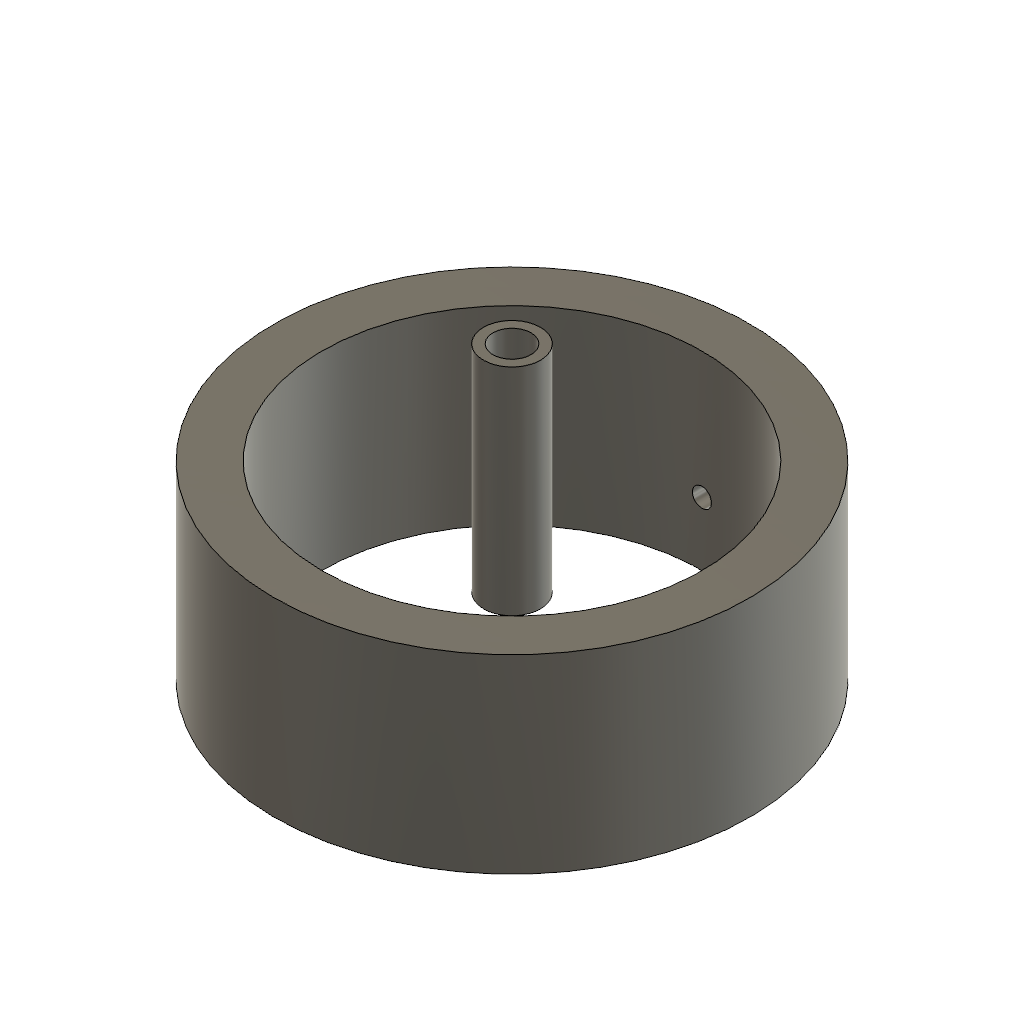
race tank (Autodesk Fusion 360 archive; units mm, degrees)
design "whel"
part number: 2026-05-14-16-49-29-881
Autodesk Fusion 360 part; units mm, degrees
sketch "Sketch1" plane through (0, 0, 0) normal (0, 1, 0) x (1, 0, 0)
  circle A0 centre (-9.0763, 7.4879) radius 42.5
  circle A1 centre (-9.0763, 7.4879) radius 30.0076
  line L0 (-13.6697, 40) -> (-4.7657, 40)
  line L1 (-4.7657, 40) -> (-4.7657, -24.506)
  line L2 (-4.7657, -24.506) -> (-13.6697, -24.506)
  line L3 (-13.6697, -24.506) -> (-13.6697, 40)
  line L4 (-41, 12.6264) -> (22, 12.6264)
  line L5 (22, 12.6264) -> (22, 3.3132)
  line L6 (22, 3.3132) -> (-41, 3.3132)
  line L7 (-41, 3.3132) -> (-41, 12.6264)
  line L8 (-9.0763, 7.4879) -> (-12.1102, 10.0947)
  line L9 (-9.0763, 7.4879) -> (-6.0424, 4.8812)
  line L10 (-12.1102, 10.0947) -> (-31.4914, -12.4624)
  line L11 (-6.0424, 4.8812) -> (-25.4235, -17.676)
  line L12 (-6.0424, 4.8812) -> (13.3388, 27.4383)
  line L13 (-12.1102, 10.0947) -> (7.2709, 32.6518)
  line L14 (-9.0763, 7.4879) -> (-6.4695, 10.5219)
  line L15 (-6.4695, 10.5219) -> (-29.0267, 29.903)
  line L16 (-6.4695, 10.5219) -> (16.0876, -8.8593)
  line L17 (-11.6831, 4.454) -> (10.8741, -14.9272)
  line L18 (-11.6831, 4.454) -> (-34.2402, 23.8352)
  dimension "d1" = 85
  dimension "d3" = 4
  dimension "d4" = 4
  dimension "d5" = 4
  dimension "d6" = 4
  constraint concentric A0 A1
  constraint horizontal L0
  constraint vertical L1
  constraint horizontal L2
  constraint vertical L3
  constraint horizontal L4
  constraint vertical L5
  constraint horizontal L6
  constraint vertical L7
  constraint coincident A0.centre A1.centre
  constraint parallel L8 L9
  constraint coincident A1 L10.end
  constraint perpendicular L8 L10
  constraint coincident A1 L11.end
  constraint perpendicular L9 L11
  constraint coincident A1 L12.end
  constraint perpendicular L9 L12
  constraint coincident A1 L13.end
  constraint perpendicular L8 L13
  constraint perpendicular L9 L14
  constraint coincident A1 L15.end
  constraint perpendicular L13 L15
  constraint coincident A1 L16.end
  constraint perpendicular L12 L16
  constraint coincident A1 L17.end
  constraint perpendicular L11 L17
  constraint coincident A1 L18.end
  measures "d1" diameter of A0
  measures "d3" distance of A0.centre L8.end
  measures "d4" distance of A0.centre L9.end
  measures "d5" distance of A0.centre L17.start
  measures "d6" distance of A0.centre L14.end
extrude "Extrude1" add sketch "Sketch1" along normal blind 40 contours A0 | A1 L1 L4 L12 L13 | A1 L4 L5 L6 | A1 L4 L6 L12 L16 | L1 L4 L12 L16 | A1 L1 L3 L13 L15 | A1 L0 L1 L3 | L1 L4 L13 L15 | L1 L4 L15 L16 | L1 L6 L12 L16 | L1 L12 L16 | L4 L13 L15 | L3 L4 L13 L15 | L1 L9 L12 L14 L16 | L4 L8 L13 L14 L15 | L1 L6 L11 L12 | A1 L1 L6 L16 L17 | A1 L3 L4 L15 L18 | L3 L4 L10 L13 | L1 L6 L11 L17 | L3 L6 L8 L9 L10 L11 L17 L18 | L3 L4 L10 L18 | A1 L1 L3 L11 L17 | L6 L11 L17 | A1 L4 L6 L10 L18 | A1 L4 L6 L7 | L3 L10 L18 | A1 L1 L2 L3 | L3 L6 L11 L17 | L3 L6 L17 L18 | L3 L6 L10 L18 | A1 L3 L6 L10 L11 makes body 1
sketch "Sketch2" plane through (0, 40, 0) normal (0, 1, 0) x (-1, 0, 0)
  circle A0 centre (9.0763, -7.4879) radius 42.5
  line L0 (-20.4881, -12.6264) -> (-0.6123, -12.6264)
  line L1 (-0.6123, -12.6264) -> (-13.3388, -27.4383)
  arc A1 (-20.4881, -12.6264) -> (-13.3388, -27.4383) centre (9.0763, -7.4879) ccw
  line L2 (-1.9204, -3.3132) -> (-20.6395, -3.3132)
  arc A2 (-16.0876, 8.8593) -> (-20.6395, -3.3132) centre (9.0763, -7.4879) ccw
  line L3 (-16.0876, 8.8593) -> (-1.9204, -3.3132)
  line L4 (4.7657, -18.6428) -> (4.7657, -37.1843)
  arc A3 (-7.2709, -32.6518) -> (4.7657, -37.1843) centre (9.0763, -7.4879) ccw
  line L5 (-7.2709, -32.6518) -> (4.7657, -18.6428)
  line L6 (13.6697, -37.1419) -> (13.6697, -16.7083)
  line L7 (13.6697, -16.7083) -> (29.0267, -29.903)
  arc A4 (13.6697, -37.1419) -> (29.0267, -29.903) centre (9.0763, -7.4879) ccw
  line L8 (21.1946, -12.6264) -> (38.6406, -12.6264)
  arc A5 (34.2402, -23.8352) -> (38.6406, -12.6264) centre (9.0763, -7.4879) ccw
  line L9 (34.2402, -23.8352) -> (21.1946, -12.6264)
  line L10 (13.6697, 3.996) -> (13.6697, 22.166)
  arc A6 (25.4235, 17.676) -> (13.6697, 22.166) centre (9.0763, -7.4879) ccw
  line L11 (25.4235, 17.676) -> (13.6697, 3.996)
  line L12 (4.7657, 22.2084) -> (4.7657, 1.4894)
  line L13 (4.7657, 1.4894) -> (-10.8741, 14.9272)
  arc A7 (4.7657, 22.2084) -> (-10.8741, 14.9272) centre (9.0763, -7.4879) ccw
  line L14 (38.792, -3.3132) -> (17.9369, -3.3132)
  line L15 (17.9369, -3.3132) -> (31.4914, 12.4624)
  arc A8 (38.792, -3.3132) -> (31.4914, 12.4624) centre (9.0763, -7.4879) ccw
  circle A9 centre (9.0763, -7.4879) radius 30.0076
  constraint concentric A0 A9
extrude "Extrude2" cut sketch "Sketch2" against normal blind 10 contours L0 L1 L2 L3 L4 L5 L6 L7 L8 L9 L10 L11 L12 L13 L14 L15 A9 bodies 1
sketch "Sketch3" plane through (0, 30, 0) normal (0, 1, 0) x (-1, 0, 0)
  arc A0 (38.6406, -12.6264) -> (38.792, -3.3132) centre (9.0763, -7.4879) ccw
  line L0 (38.792, -3.3132) -> (17.9369, -3.3132)
  line L1 (17.9369, -3.3132) -> (31.4914, 12.4624)
  arc A1 (31.4914, 12.4624) -> (25.4235, 17.676) centre (9.0763, -7.4879) ccw
  line L2 (25.4235, 17.676) -> (13.6697, 3.996)
  line L3 (13.6697, 3.996) -> (13.6697, 22.166)
  arc A2 (13.6697, 22.166) -> (4.7657, 22.2084) centre (9.0763, -7.4879) ccw
  line L4 (4.7657, 22.2084) -> (4.7657, 1.4894)
  line L5 (4.7657, 1.4894) -> (-10.8741, 14.9272)
  arc A3 (-10.8741, 14.9272) -> (-16.0876, 8.8593) centre (9.0763, -7.4879) ccw
  line L6 (-16.0876, 8.8593) -> (-1.9204, -3.3132)
  line L7 (-1.9204, -3.3132) -> (-20.6395, -3.3132)
  arc A4 (-20.6395, -3.3132) -> (-20.4881, -12.6264) centre (9.0763, -7.4879) ccw
  line L8 (-20.4881, -12.6264) -> (-0.6123, -12.6264)
  line L9 (-0.6123, -12.6264) -> (-13.3388, -27.4383)
  arc A5 (-13.3388, -27.4383) -> (-7.2709, -32.6518) centre (9.0763, -7.4879) ccw
  line L10 (-7.2709, -32.6518) -> (4.7657, -18.6428)
  line L11 (4.7657, -18.6428) -> (4.7657, -37.1843)
  arc A6 (4.7657, -37.1843) -> (13.6697, -37.1419) centre (9.0763, -7.4879) ccw
  line L12 (13.6697, -37.1419) -> (13.6697, -16.7083)
  line L13 (13.6697, -16.7083) -> (29.0267, -29.903)
  arc A7 (29.0267, -29.903) -> (34.2402, -23.8352) centre (9.0763, -7.4879) ccw
  line L14 (34.2402, -23.8352) -> (21.1946, -12.6264)
  line L15 (21.1946, -12.6264) -> (38.6406, -12.6264)
  circle A8 centre (9.0763, -7.4879) radius 6
  dimension "d11" = 12
  constraint concentric A0 A8
  measures "d11" diameter of A8
extrude "Extrude3" add sketch "Sketch3" along normal blind 20 contours A8 bodies 1
sketch "Sketch4" plane through (0, 50, 0) normal (0, 1, 0) x (-1, 0, 0)
  circle A0 centre (9.0763, -7.4879) radius 6
  circle A1 centre (9.0763, -7.4879) radius 3
  dimension "d14" = 6
  constraint concentric A0 A1
  measures "d14" diameter of A1
extrude "Extrude4" cut sketch "Sketch4" against normal blind 40 contours A1 bodies 1
move_face "MoveFace1" by (0, -10, 0) 1 faces at (-13.9891, 50, -8.2059) on bodies 1
move_face "MoveFace2" by (0, 10, 0) 1 faces at (-5.941, 0, -9.2817) on bodies 1
sketch "Sketch5" plane through (0, 10, 0) normal (0, -1, 0) x (1, 0, 0)
  line L0 (-17.9369, -3.3132) -> (-38.792, -3.3132)
  arc A0 (-31.4914, 12.4624) -> (-38.792, -3.3132) centre (-9.0763, -7.4879) ccw
  line L1 (-31.4914, 12.4624) -> (-17.9369, -3.3132)
  line L2 (-4.7657, 1.4894) -> (-4.7657, 22.2084)
  arc A1 (10.8741, 14.9272) -> (-4.7657, 22.2084) centre (-9.0763, -7.4879) ccw
  line L3 (10.8741, 14.9272) -> (-4.7657, 1.4894)
  line L4 (-13.6697, 22.166) -> (-13.6697, 3.996)
  line L5 (-13.6697, 3.996) -> (-25.4235, 17.676)
  arc A2 (-13.6697, 22.166) -> (-25.4235, 17.676) centre (-9.0763, -7.4879) ccw
  line L6 (-38.6406, -12.6264) -> (-21.1946, -12.6264)
  line L7 (-21.1946, -12.6264) -> (-34.2402, -23.8352)
  arc A3 (-38.6406, -12.6264) -> (-34.2402, -23.8352) centre (-9.0763, -7.4879) ccw
  line L8 (-13.6697, -16.7083) -> (-13.6697, -37.1419)
  arc A4 (-29.0267, -29.903) -> (-13.6697, -37.1419) centre (-9.0763, -7.4879) ccw
  line L9 (-29.0267, -29.903) -> (-13.6697, -16.7083)
  line L10 (-4.7657, -37.1843) -> (-4.7657, -18.6428)
  line L11 (-4.7657, -18.6428) -> (7.2709, -32.6518)
  arc A5 (-4.7657, -37.1843) -> (7.2709, -32.6518) centre (-9.0763, -7.4879) ccw
  line L12 (20.6395, -3.3132) -> (1.9204, -3.3132)
  line L13 (1.9204, -3.3132) -> (16.0876, 8.8593)
  arc A6 (20.6395, -3.3132) -> (16.0876, 8.8593) centre (-9.0763, -7.4879) ccw
  line L14 (0.6123, -12.6264) -> (20.4881, -12.6264)
  arc A7 (13.3388, -27.4383) -> (20.4881, -12.6264) centre (-9.0763, -7.4879) ccw
  line L15 (13.3388, -27.4383) -> (0.6123, -12.6264)
  circle A8 centre (-9.0763, -7.4879) radius 42.5
  circle A9 centre (-9.0763, -7.4879) radius 3
  circle A10 centre (-9.0763, -7.4879) radius 3
  circle A11 centre (-9.0763, -7.4879) radius 4.5
  dimension "d17" = 9
  constraint concentric A0 A10
  constraint concentric A0 A11
  measures "d17" diameter of A11
extrude "Extrude5" add sketch "Sketch5" along normal blind 10 separate body contours A11 makes body 2
sketch "Sketch6" plane through (0, 0, 0) normal (0, -1, 0) x (1, 0, 0)
  circle A0 centre (-9.0763, -7.4879) radius 3
  circle A1 centre (-9.0763, -7.4879) radius 4.5
  circle A2 centre (-9.0763, -7.4879) radius 4.5
  constraint concentric A0 A2
sketch "Sketch7" plane through (-2.7602, 0, 3.2125) normal (-0.651692, 0, 0.758484) x (0.758484, 0, 0.651692)
  line L0 (17.9757, 30) -> (-2.644, 30)
  line L1 (-2.644, 30) -> (-2.644, 10)
  line L2 (-2.644, 10) -> (17.9757, 10)
  line L3 (17.9757, 10) -> (17.9757, 30)
  line L4 (-11.7599, 0) -> (-11.7599, 6.7)
  line L5 (-11.7599, 0) -> (-11.7599, 9.4)
  line L6 (-11.7599, 6.7) -> (-11.7599, 8.05)
  line L7 (-11.7599, 0) -> (-11.7599, 10)
  circle A0 centre (-11.7599, 10) radius 1.5
  dimension "d21" = 6.7
  dimension "d22" = 9.4
  dimension "d23" = 1.35
  dimension "d34" = 3
  constraint parallel L4 L5
  constraint parallel L5 L6
  constraint parallel L5 L7
  constraint coincident L7.end A0.centre
  measures "d21" distance of L4.start L4.end
  measures "d22" distance of L4.start L5.end
  measures "d23" distance of L4.end L6.end
  measures "d34" diameter of A0
sketch "Sketch10" plane through (0, 10, 0) normal (0, -1, 0) x (1, 0, 0)
  circle A0 centre (-9.0763, -7.4879) radius 3
  circle A1 centre (-9.0763, -7.4879) radius 42.5
  line L0 (0.6123, -12.6264) -> (20.4881, -12.6264)
  arc A2 (13.3388, -27.4383) -> (20.4881, -12.6264) centre (-9.0763, -7.4879) ccw
  line L1 (13.3388, -27.4383) -> (0.6123, -12.6264)
  line L2 (20.6395, -3.3132) -> (1.9204, -3.3132)
  line L3 (1.9204, -3.3132) -> (16.0876, 8.8593)
  arc A3 (20.6395, -3.3132) -> (16.0876, 8.8593) centre (-9.0763, -7.4879) ccw
  line L4 (-4.7657, -37.1843) -> (-4.7657, -18.6428)
  line L5 (-4.7657, -18.6428) -> (7.2709, -32.6518)
  arc A4 (-4.7657, -37.1843) -> (7.2709, -32.6518) centre (-9.0763, -7.4879) ccw
  line L6 (-13.6697, -16.7083) -> (-13.6697, -37.1419)
  arc A5 (-29.0267, -29.903) -> (-13.6697, -37.1419) centre (-9.0763, -7.4879) ccw
  line L7 (-29.0267, -29.903) -> (-13.6697, -16.7083)
  line L8 (-38.6406, -12.6264) -> (-21.1946, -12.6264)
  line L9 (-21.1946, -12.6264) -> (-34.2402, -23.8352)
  arc A6 (-38.6406, -12.6264) -> (-34.2402, -23.8352) centre (-9.0763, -7.4879) ccw
  line L10 (-13.6697, 22.166) -> (-13.6697, 3.996)
  line L11 (-13.6697, 3.996) -> (-25.4235, 17.676)
  arc A7 (-13.6697, 22.166) -> (-25.4235, 17.676) centre (-9.0763, -7.4879) ccw
  line L12 (-4.7657, 1.4894) -> (-4.7657, 22.2084)
  arc A8 (10.8741, 14.9272) -> (-4.7657, 22.2084) centre (-9.0763, -7.4879) ccw
  line L13 (10.8741, 14.9272) -> (-4.7657, 1.4894)
  line L14 (-17.9369, -3.3132) -> (-38.792, -3.3132)
  arc A9 (-31.4914, 12.4624) -> (-38.792, -3.3132) centre (-9.0763, -7.4879) ccw
  line L15 (-31.4914, 12.4624) -> (-17.9369, -3.3132)
  circle A10 centre (-9.0763, -7.4879) radius 30.0076
  circle A11 centre (-9.0763, -7.4879) radius 4.5
  dimension "d35" = 9
  constraint concentric A0 A10
  constraint concentric A10 A11
  measures "d35" diameter of A11
extrude "Extrude9" cut sketch "Sketch10" against normal blind 5 contours L0 L1 L2 L3 L4 L5 L6 L7 L8 L9 L10 L11 L12 L13 L14 L15 A10 bodies 1
move_face "MoveFace5" by (0, -10, 0) 1 faces at (-20.3324, 10, -44.0512) on bodies 1
extrude "Extrude10" cut sketch "Sketch7" against normal blind 56 contours A0 bodies 1 2
move_face "MoveFace6" by (0, -10, 0) 1 faces at (-13.9891, 40, -6.77) on bodies 1
move_face "MoveFace7" by (0, -10, 0) 1 faces at (-47.329, 40, -7.4879) on bodies 1
sketch "Sketch11" plane through (0, 30, 0) normal (0, 1, 0) x (-1, 0, 0)
  arc A0 (-16.0876, 8.8593) -> (-20.6395, -3.3132) centre (9.0763, -7.4879) ccw
  line L0 (-16.0876, 8.8593) -> (-1.9204, -3.3132)
  line L1 (-1.9204, -3.3132) -> (-20.6395, -3.3132)
  line L2 (-7.2709, -32.6518) -> (4.7657, -18.6428)
  line L3 (4.7657, -18.6428) -> (4.7657, -37.1843)
  arc A1 (-7.2709, -32.6518) -> (4.7657, -37.1843) centre (9.0763, -7.4879) ccw
  line L4 (13.6697, -37.1419) -> (13.6697, -16.7083)
  line L5 (13.6697, -16.7083) -> (29.0267, -29.903)
  arc A2 (13.6697, -37.1419) -> (29.0267, -29.903) centre (9.0763, -7.4879) ccw
  line L6 (34.2402, -23.8352) -> (21.1946, -12.6264)
  line L7 (21.1946, -12.6264) -> (38.6406, -12.6264)
  arc A3 (34.2402, -23.8352) -> (38.6406, -12.6264) centre (9.0763, -7.4879) ccw
  line L8 (38.792, -3.3132) -> (17.9369, -3.3132)
  line L9 (17.9369, -3.3132) -> (31.4914, 12.4624)
  arc A4 (38.792, -3.3132) -> (31.4914, 12.4624) centre (9.0763, -7.4879) ccw
  line L10 (25.4235, 17.676) -> (13.6697, 3.996)
  line L11 (13.6697, 3.996) -> (13.6697, 22.166)
  arc A5 (25.4235, 17.676) -> (13.6697, 22.166) centre (9.0763, -7.4879) ccw
  line L12 (4.7657, 22.2084) -> (4.7657, 1.4894)
  line L13 (4.7657, 1.4894) -> (-10.8741, 14.9272)
  arc A6 (4.7657, 22.2084) -> (-10.8741, 14.9272) centre (9.0763, -7.4879) ccw
  circle A7 centre (9.0763, -7.4879) radius 42.5
  line L14 (-20.4881, -12.6264) -> (-0.6123, -12.6264)
  line L15 (-0.6123, -12.6264) -> (-13.3388, -27.4383)
  arc A8 (-20.4881, -12.6264) -> (-13.3388, -27.4383) centre (9.0763, -7.4879) ccw
  circle A9 centre (9.0763, -7.4879) radius 3
  circle A10 centre (9.0763, -7.4879) radius 30
  circle A11 centre (9.0763, -7.4879) radius 4.5
  dimension "d40" = 60
  dimension "d41" = 9
  constraint concentric A0 A10
  constraint concentric A0 A11
  measures "d40" diameter of A10
  measures "d41" diameter of A11
extrude "Extrude11" cut sketch "Sketch11" against normal blind 6 contours L0 L1 L2 L3 L4 L5 L6 L7 L8 L9 L10 L11 L12 L13 L14 L15 A10 bodies 1
sketch "Sketch12" plane through (0, 0, 0) normal (0, -1, 0) x (1, 0, 0)
  circle A0 centre (-9.0763, -7.4879) radius 30.0076
  circle A1 centre (-9.0763, -7.4879) radius 42.5
  circle A2 centre (-9.0763, -7.4879) radius 37.5
  circle A3 centre (-9.0763, -7.4879) radius 42.5
  dimension "d44" = 75
  dimension "d45" = 85
  constraint concentric A0 A2
  constraint concentric A0 A3
  measures "d44" diameter of A2
  measures "d45" diameter of A3
extrude "Extrude12" cut sketch "Sketch12" against normal blind 40 contours A1 A3 bodies 1
sketch "Sketch13" plane through (0, 0, 0) normal (0, -1, 0) x (1, 0, 0)
  circle A0 centre (-9.0763, -7.4879) radius 3
  circle A1 centre (-9.0763, -7.4879) radius 4.5
  circle A2 centre (-9.0763, -7.4879) radius 3.025
  dimension "d48" = 6.05
  constraint concentric A0 A2
  measures "d48" diameter of A2
move_body "Move1" bodies 1 2 to x (0.758362, 0, -0.651834) y (0, 1, 0) z (0.651834, 0, 0.758362) at (18.0701, 0, -41.2308)
sketch "Sketch14" plane through (-0.0069, 0, -36.9919) normal (-0.000187, 0, -1) x (-1, 0, 0.000187)
  line L0 (-4.8179, 10) -> (-7.8179, 10)
  arc A0 (-7.8179, 10) -> (-4.8179, 10) centre (-6.3179, 10) ccw
  circle A1 centre (-6.3179, 10) radius 2.3282
  constraint concentric A0 A1
extrude "Extrude13" cut 1 faces at (-5.8112, 15, -29.1666) along direction (0, 1, 0) blind 21 on bodies 1 bodies 1 makes body 3 at (4.4027, 16.7321, -45.0708)
extrude "Extrude14" add 1 faces at (9.3278, 30, -43.5904) along direction (0, 1, 0) blind 16 on bodies 3 bodies 3
extrude "Extrude15" cut 1 faces at (6.5026, 0, -37.0082) along direction (0, 1, 0) blind 22 on bodies 2 bodies 2 3
extrude "Extrude16" add 1 faces at (3.2859, 22, -38.3973) along direction (0, -1, 0) blind 10 on bodies 3 bodies 2 3
equation "d48 = 6.000 mm + 0.05 mm"

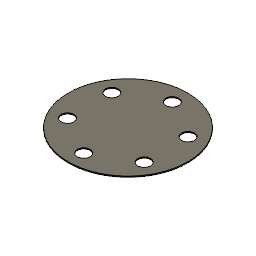
design "tempo"
part number: 2026-05-15-12-56-36-307
Autodesk Fusion 360 part; units mm, degrees
sketch "Sketch1" plane through (0, 0, 0) normal (0, 1, 0) x (1, 0, 0)
  circle A0 centre (0, 0) radius 23.5
  dimension "d1" = 47
  constraint coincident A0.centre origin
  measures "d1" diameter of A0
extrude "Extrude1" add sketch "Sketch1" along normal blind 0.4
sketch "Sketch2" plane through (0, 0.4, 0) normal (0, 1, 0) x (-1, 0, 0)
  circle A0 centre (0, 0) radius 23.5
  line L0 (-16.617, 16.617) -> (-14.0856, 14.0856)
  line L1 (-14.0856, 14.0856) -> (-12.3178, 12.3178)
  line L2 (-16.617, -16.617) -> (-12.3178, -12.3178)
  line L3 (16.617, 16.617) -> (12.3178, 12.3178)
  line L4 (16.617, -16.617) -> (12.3178, -12.3178)
  line L5 (0, 23.5) -> (0, 17.42)
  circle A1 centre (0, 17.42) radius 2.5
  line L6 (0, -23.5) -> (0, -17.42)
  circle A2 centre (0, -17.42) radius 2.5
  line L7 (0, 0) -> (23.3804, 0) construction
  line L8 (0, 0) -> (23.4036, 0) construction
  line L9 (0, 0) -> (12, 0) construction
  line L10 (0, 0) -> (23.4493, 0) construction
  line L11 (-20.248, -11.6902) -> (-14.9826, -8.6502)
  circle A3 centre (-14.9826, -8.6502) radius 2.5
  line L12 (-20.2681, 11.7018) -> (-15.0027, 8.6618)
  circle A4 centre (-15.0027, 8.6618) radius 2.5
  line L13 (20.3516, 11.75) -> (15.0862, 8.71)
  circle A5 centre (15.0862, 8.71) radius 2.5
  line L14 (20.3077, -11.7246) -> (15.0422, -8.6846)
  circle A6 centre (15.0422, -8.6846) radius 2.5
  dimension "d6" = 3.58
  dimension "d7" = 2.5
  dimension "d9" = 6.08
  dimension "d11" = 6.08
  dimension "d13" = 6.08
  dimension "d15" = 6.08
  dimension "d16" = 5
  dimension "d17" = 6.08
  dimension "d18" = 5
  dimension "d26" = 6.08
  dimension "d27" = 5
  dimension "d28" = 6.08
  dimension "d29" = 5
  dimension "d30" = 6.08
  dimension "d31" = 5
  dimension "d32" = 6.08
  dimension "d33" = 5
  constraint coincident A0 L0.start
  constraint coincident A0 L3.start
  constraint coincident A0 L6.start
  constraint coincident A0 L5.start
  constraint coincident L5.end A1.centre
  constraint coincident L6.end A2.centre
  constraint horizontal L7
  constraint coincident A0.centre L7.start
  constraint horizontal L8
  constraint horizontal L9
  constraint horizontal L10
  constraint coincident L11.end A3.centre
  constraint coincident L12.end A4.centre
  constraint coincident A0 L13.start
  constraint coincident L13.end A5.centre
  constraint coincident L14.end A6.centre
  measures "d6" distance of L0.start L0.end
  measures "d7" distance of L0.end L1.end
  measures "d9" distance of L2.start L2.end
  measures "d11" distance of L3.start L3.end
  measures "d13" distance of L4.start L4.end
  measures "d15" distance of L5.start L5.end
  measures "d16" diameter of A1
  measures "d17" distance of L6.start L6.end
  measures "d18" diameter of A2
  measures "d26" distance of L11.start L11.end
  measures "d27" diameter of A3
  measures "d28" distance of L12.start L12.end
  measures "d29" diameter of A4
  measures "d30" distance of L13.start L13.end
  measures "d31" diameter of A5
  measures "d32" distance of L14.start L14.end
  measures "d33" diameter of A6
extrude "Extrude2" cut sketch "Sketch2" against normal blind 10 contours A1 | A2 | A3 | A4 | A5 | A6
equation "d9 = 3.58 mm + 2.5 mm"
equation "d11 = 3.58 mm + 2.5 mm"
equation "d13 = 3.58 mm + 2.5 mm"
equation "d15 = 3.58 mm + 2.5 mm"
equation "d17 = 3.58 mm + 2.5 mm"

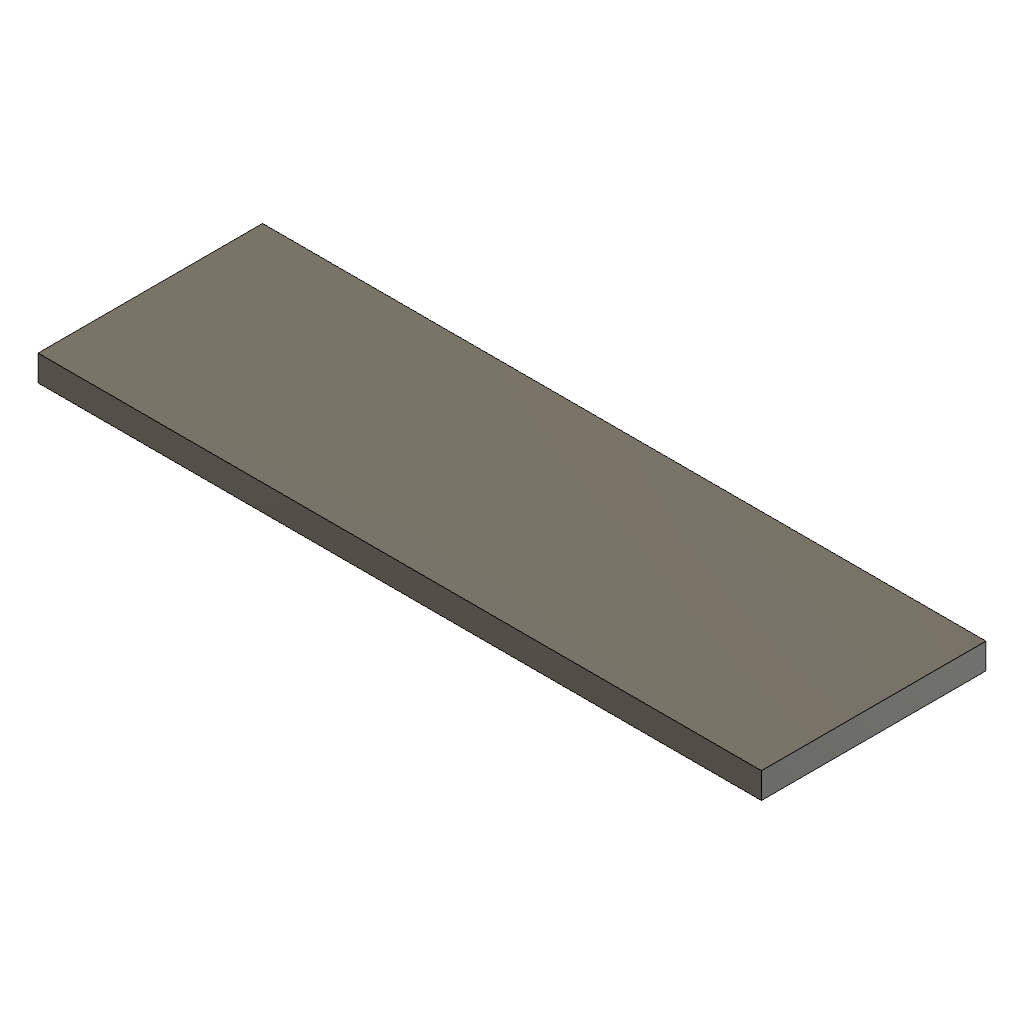
design "c"
part number: 2026-09-22-14-13-15-717
Autodesk Fusion 360 part; units mm, degrees
other "DerivedContext1"
sketch "sketch 241" plane through (0, 0, 0) normal (0, 1, 0) x (1, 0, 0)
  line L0 (-39.2615, 186.6944) -> (240, 186.6944)
  line L1 (240, 186.6944) -> (240, 100)
  line L2 (240, 100) -> (-39.2615, 100)
  line L3 (-39.2615, 100) -> (-39.2615, 186.6944)
extrude "Extrude1" add sketch "sketch 241" along normal blind 10
